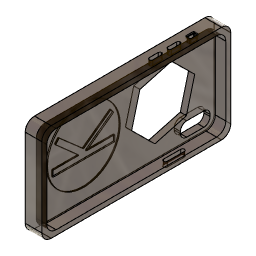
Mitt Mobildeksel (Autodesk Fusion 360 design; units mm, degrees)
Autodesk Fusion 360 part; units mm, degrees
sketch "Sketch1" plane through (0, 0, 0) normal (1, 0, 0) x (0, 1, 0)
  line L0 (76.5, 39.5) -> (-76.5, 39.5)
  line L1 (-76.5, 39.5) -> (-76.5, -39.5)
  line L2 (-76.5, -39.5) -> (76.5, -39.5)
  line L3 (76.5, -39.5) -> (76.5, 39.5)
  line L4 (76.5, 39.5) -> (-76.5, -39.5) construction
  line L5 (-76.5, 39.5) -> (76.5, -39.5) construction
  dimension "d6" = 153
  dimension "d7" = 79
  constraint horizontal L0
  constraint perpendicular L0 L1
  constraint parallel L0 L2
  constraint parallel L1 L3
  constraint coincident L4 origin
  constraint coincident L5 origin
  measures "d6" distance of L1.end L2.end
  measures "d7" distance of L0.end L1.end
extrude "Extrude1" add sketch "Sketch1" along normal blind 13.5
sketch "Sketch2" plane through (0, 0, 0) normal (1, 0, 0) x (0, 1, 0)
sketch "Sketch3" plane through (13.5, 0, 0) normal (1, 0, 0) x (0, 1, 0)
  line L0 (76.5, -39.5) -> (76.5, 39.5)
  line L1 (76.5, 39.5) -> (-76.5, 39.5)
  line L2 (-76.5, 39.5) -> (-76.5, -39.5)
  line L3 (-76.5, -39.5) -> (76.5, -39.5)
  line L4 (72.5, 35.5) -> (-72.5, 35.5)
  line L5 (-72.5, 35.5) -> (-72.5, -35.5)
  line L6 (-72.5, -35.5) -> (72.5, -35.5)
  line L7 (72.5, -35.5) -> (72.5, 35.5)
  line L8 (72.5, 35.5) -> (-72.5, -35.5) construction
  line L9 (-72.5, 35.5) -> (72.5, -35.5) construction
  dimension "d10" = 145
  dimension "d11" = 71
  constraint horizontal L4
  constraint perpendicular L4 L5
  constraint parallel L4 L6
  constraint parallel L5 L7
  constraint coincident L8 origin
  constraint coincident L9 origin
  measures "d10" distance of L5.end L6.end
  measures "d11" distance of L4.end L5.end
extrude "Extrude2" cut sketch "Sketch3" against normal blind 8.5 contours L4 L5 L6 L7
fillet "Fillet1" radius 7.5 4 edges at (6.75, -76.5, 39.5) (6.75, 76.5, 39.5) (6.75, -76.5, -39.5) (6.75, 76.5, -39.5)
fillet "Fillet2" radius 7.5 4 edges at (9.25, -72.5, 35.5) (9.25, 72.5, -35.5) (9.25, 72.5, 35.5) (9.25, -72.5, -35.5)
sketch "Sketch4" plane through (0, 0, 0) normal (-1, 0, 0) x (0, -1, 0)
  arc A0 (-76.5, -32) -> (-69, -39.5) centre (-69, -32) ccw
  line L0 (-69, -39.5) -> (69, -39.5)
  arc A1 (69, -39.5) -> (76.5, -32) centre (69, -32) ccw
  line L1 (76.5, -32) -> (76.5, 32)
  arc A2 (76.5, 32) -> (69, 39.5) centre (69, 32) ccw
  line L2 (69, 39.5) -> (-69, 39.5)
  arc A3 (-69, 39.5) -> (-76.5, 32) centre (-69, 32) ccw
  line L3 (-76.5, 32) -> (-76.5, -32)
  line L4 (-44.2147, -20.46) -> (-68.2147, -20.46)
  line L5 (-68.2147, -20.46) -> (-68.2147, -31.96)
  line L6 (-68.2147, -31.96) -> (-44.2147, -31.96)
  line L7 (-44.2147, -31.96) -> (-44.2147, -20.46)
  line L8 (-44.2147, -20.46) -> (-68.2147, -31.96) construction
  line L9 (-68.2147, -20.46) -> (-44.2147, -31.96) construction
  point P0 (-56.2147, -26.21)
  dimension "d16" = 24
  dimension "d17" = 11.5
  constraint horizontal L4
  constraint perpendicular L4 L5
  constraint parallel L4 L6
  constraint parallel L5 L7
  constraint coincident L8 P0
  constraint coincident L9 P0
  measures "d16" distance of L5.end L6.end
  measures "d17" distance of L4.end L5.end
extrude "Extrude3" cut sketch "Sketch4" against normal blind 20 contours L4 L5 L6 L7
fillet "Fillet3" radius 5 4 edges at (2.5, 44.2147, -20.46) (2.5, 68.2147, -20.46) (2.5, 44.2147, -31.96) (2.5, 68.2147, -31.96)
sketch "Sketch5" plane through (0, 0, -35.5) normal (0, 0, 1) x (-1, 0, 0)
  line L0 (-5, 65) -> (-13.5, 65)
  line L1 (-13.5, 65) -> (-13.5, -65)
  line L2 (-13.5, -65) -> (-5, -65)
  line L3 (-5, -65) -> (-5, 65)
  line L4 (-7.5, -26.5) -> (-10.5, -26.5)
  line L5 (-10.5, -26.5) -> (-10.5, -43.5)
  line L6 (-10.5, -43.5) -> (-7.5, -43.5)
  line L7 (-7.5, -43.5) -> (-7.5, -26.5)
  line L8 (-7.5, -26.5) -> (-10.5, -43.5) construction
  line L9 (-10.5, -26.5) -> (-7.5, -43.5) construction
  point P0 (-9, -35)
  dimension "d21" = 3
  dimension "d22" = 17
  constraint horizontal L4
  constraint perpendicular L4 L5
  constraint parallel L4 L6
  constraint parallel L5 L7
  constraint coincident L8 P0
  constraint coincident L9 P0
  measures "d21" distance of L5.end L6.end
  measures "d22" distance of L4.end L5.end
extrude "Extrude4" cut sketch "Sketch5" against normal blind 6 contours L4 L5 L6 L7
fillet "Fillet4" radius 1.5 4 edges at (7.5, 26.5, -37.5) (10.5, 26.5, -37.5) (7.5, 43.5, -37.5) (10.5, 43.5, -37.5)
sketch "Sketch6" plane through (0, 0, 39.5) normal (0, 0, 1) x (-1, 0, 0)
  line L0 (-13.5, -69) -> (0, -69)
  line L1 (0, -69) -> (0, 69)
  line L2 (0, 69) -> (-13.5, 69)
  line L3 (-13.5, 69) -> (-13.5, -69)
  line L4 (-8.5982, -48.5986) -> (-5.5982, -48.5986)
  line L5 (-5.5982, -48.5986) -> (-5.5982, -54.5986)
  line L6 (-5.5982, -54.5986) -> (-8.5982, -54.5986)
  line L7 (-8.5982, -54.5986) -> (-8.5982, -48.5986)
  line L8 (-8.5982, -48.5986) -> (-5.5982, -54.5986) construction
  line L9 (-5.5982, -48.5986) -> (-8.5982, -54.5986) construction
  point P0 (-7.0982, -51.5986)
  dimension "d26" = 3
  dimension "d27" = 6
  constraint horizontal L4
  constraint perpendicular L4 L5
  constraint parallel L4 L6
  constraint parallel L5 L7
  constraint coincident L8 P0
  constraint coincident L9 P0
  measures "d26" distance of L5.end L6.end
  measures "d27" distance of L4.end L5.end
extrude "Extrude5" cut sketch "Sketch6" against normal blind 5 contours L4 L5 L6 L7
sketch "Sketch7" plane through (0, 0, 39.5) normal (0, 0, 1) x (-1, 0, 0)
  line L0 (-5.5982, -48.5986) -> (-5.5982, -54.5986)
  line L1 (-5.5982, -54.5986) -> (-8.5982, -54.5986)
  line L2 (-8.5982, -54.5986) -> (-8.5982, -48.5986)
  line L3 (-8.5982, -48.5986) -> (-5.5982, -48.5986)
  line L4 (-13.5, -69) -> (0, -69)
  line L5 (0, -69) -> (0, 69)
  line L6 (0, 69) -> (-13.5, 69)
  line L7 (-13.5, 69) -> (-13.5, -69)
  line L8 (-9, -48.3) -> (-5, -48.3)
  line L9 (-5, -48.3) -> (-5, -54.9)
  line L10 (-5, -54.9) -> (-9, -54.9)
  line L11 (-9, -54.9) -> (-9, -48.3)
  line L12 (-9, -48.3) -> (-5, -54.9) construction
  line L13 (-5, -48.3) -> (-9, -54.9) construction
  point P0 (-7, -51.6)
  constraint horizontal L8
  constraint perpendicular L8 L9
  constraint parallel L8 L10
  constraint parallel L9 L11
  constraint coincident L12 P0
  constraint coincident L13 P0
extrude "Extrude6" cut sketch "Sketch7" against normal blind 1 contours L8 L9 L10 L11
fillet "Fillet5" radius 0.5 4 edges at (5.5982, 54.5986, 37) (8.5982, 48.5986, 37) (5.5982, 48.5986, 37) (8.5982, 54.5986, 37)
fillet "Fillet6" radius 0.5 4 edges at (9, 54.9, 39) (9, 48.3, 39) (5, 48.3, 39) (5, 54.9, 39)
sketch "Sketch8" plane through (0, 0, 39.5) normal (0, 0, 1) x (-1, 0, 0)
  line L0 (-5, -48.8) -> (-5, -54.4)
  arc A0 (-5.5, -54.9) -> (-5, -54.4) centre (-5.5, -54.4) ccw
  line L1 (-5.5, -54.9) -> (-8.5, -54.9)
  arc A1 (-9, -54.4) -> (-8.5, -54.9) centre (-8.5, -54.4) ccw
  line L2 (-9, -54.4) -> (-9, -48.8)
  arc A2 (-8.5, -48.3) -> (-9, -48.8) centre (-8.5, -48.8) ccw
  line L3 (-8.5, -48.3) -> (-5.5, -48.3)
  arc A3 (-5, -48.8) -> (-5.5, -48.3) centre (-5.5, -48.8) ccw
  line L4 (-13.5, -69) -> (0, -69)
  line L5 (0, -69) -> (0, 69)
  line L6 (0, 69) -> (-13.5, 69)
  line L7 (-13.5, 69) -> (-13.5, -69)
  line L8 (-5.5, -42) -> (-8.5, -42)
  line L9 (-8.5, -42) -> (-8.5, -32)
  line L10 (-8.5, -32) -> (-5.5, -32)
  line L11 (-5.5, -32) -> (-5.5, -42)
  line L12 (-5.5, -42) -> (-8.5, -32) construction
  line L13 (-8.5, -42) -> (-5.5, -32) construction
  point P0 (-7, -37)
  dimension "d34" = 3
  dimension "d35" = 10
  constraint horizontal L8
  constraint perpendicular L8 L9
  constraint parallel L8 L10
  constraint parallel L9 L11
  constraint coincident L12 P0
  constraint coincident L13 P0
  measures "d34" distance of L9.end L10.end
  measures "d35" distance of L8.end L9.end
extrude "Extrude7" cut sketch "Sketch8" against normal blind 17 contours L8 L9 L10 L11
sketch "Sketch9" plane through (0, 0, 39.5) normal (0, 0, 1) x (-1, 0, 0)
  line L0 (-8.5, -42) -> (-8.5, -32)
  line L1 (-8.5, -32) -> (-5.5, -32)
  line L2 (-5.5, -32) -> (-5.5, -42)
  line L3 (-5.5, -42) -> (-8.5, -42)
  line L4 (-5, -48.8) -> (-5, -54.4)
  arc A0 (-5.5, -54.9) -> (-5, -54.4) centre (-5.5, -54.4) ccw
  line L5 (-5.5, -54.9) -> (-8.5, -54.9)
  arc A1 (-9, -54.4) -> (-8.5, -54.9) centre (-8.5, -54.4) ccw
  line L6 (-9, -54.4) -> (-9, -48.8)
  arc A2 (-8.5, -48.3) -> (-9, -48.8) centre (-8.5, -48.8) ccw
  line L7 (-8.5, -48.3) -> (-5.5, -48.3)
  arc A3 (-5, -48.8) -> (-5.5, -48.3) centre (-5.5, -48.8) ccw
  line L8 (-13.5, -69) -> (0, -69)
  line L9 (0, -69) -> (0, 69)
  line L10 (0, 69) -> (-13.5, 69)
  line L11 (-13.5, 69) -> (-13.5, -69)
  line L12 (-8.5, -27) -> (-5.5, -27)
  line L13 (-5.5, -27) -> (-5.5, -17)
  line L14 (-5.5, -17) -> (-8.5, -17)
  line L15 (-8.5, -17) -> (-8.5, -27)
  line L16 (-8.5, -27) -> (-5.5, -17) construction
  line L17 (-5.5, -27) -> (-8.5, -17) construction
  point P0 (-7, -22)
  dimension "d38" = 3
  dimension "d39" = 10
  constraint horizontal L12
  constraint perpendicular L12 L13
  constraint parallel L12 L14
  constraint parallel L13 L15
  constraint coincident L16 P0
  constraint coincident L17 P0
  measures "d38" distance of L13.end L14.end
  measures "d39" distance of L12.end L13.end
extrude "Extrude8" cut sketch "Sketch9" against normal blind 9 contours L12 L13 L14 L15
fillet "Fillet7" radius 1.25 4 edges at (5.5, 32, 37.5) (8.5, 32, 37.5) (5.5, 42, 37.5) (8.5, 42, 37.5)
fillet "Fillet8" radius 1.25 4 edges at (8.5, 27, 37.5) (5.5, 27, 37.5) (8.5, 17, 37.5) (5.5, 17, 37.5)
form "Form1" [no effect]
sketch "Sketch10" plane through (0, 0, 0) normal (-1, 0, 0) x (0, -1, 0)
  line L0 (-63.2147, -20.46) -> (-49.2147, -20.46)
  arc A0 (-44.2147, -25.46) -> (-49.2147, -20.46) centre (-49.2147, -25.46) ccw
  line L1 (-44.2147, -25.46) -> (-44.2147, -26.96)
  arc A1 (-49.2147, -31.96) -> (-44.2147, -26.96) centre (-49.2147, -26.96) ccw
  line L2 (-49.2147, -31.96) -> (-63.2147, -31.96)
  arc A2 (-68.2147, -26.96) -> (-63.2147, -31.96) centre (-63.2147, -26.96) ccw
  line L3 (-68.2147, -26.96) -> (-68.2147, -25.46)
  arc A3 (-63.2147, -20.46) -> (-68.2147, -25.46) centre (-63.2147, -25.46) ccw
  arc A4 (-76.5, -32) -> (-69, -39.5) centre (-69, -32) ccw
  line L4 (-69, -39.5) -> (69, -39.5)
  arc A5 (69, -39.5) -> (76.5, -32) centre (69, -32) ccw
  line L5 (76.5, -32) -> (76.5, 32)
  arc A6 (76.5, 32) -> (69, 39.5) centre (69, 32) ccw
  line L6 (69, 39.5) -> (-69, 39.5)
  arc A7 (-69, 39.5) -> (-76.5, 32) centre (-69, 32) ccw
  line L7 (-76.5, 32) -> (-76.5, -32)
  line L8 (-11.3981, 20.5126) -> (-36.9638, 27.5049)
  line L9 (-36.9638, 27.5049) -> (-55.8022, 8.8605)
  line L10 (-55.8022, 8.8605) -> (-49.0748, -16.7762)
  line L11 (-49.0748, -16.7762) -> (-23.5091, -23.7685)
  line L12 (-23.5091, -23.7685) -> (-4.6707, -5.1241)
  line L13 (-4.6707, -5.1241) -> (-11.3981, 20.5126)
  point P0 (-30.2365, 1.8682)
extrude "Extrude9" cut sketch "Sketch10" against normal blind 15 contours L8 L9 L10 L11 L12 L13
sketch "Sketch11" plane through (0, 0, 0) normal (-1, 0, 0) x (0, -1, 0)
  line L0 (-36.9638, 27.5049) -> (-11.3981, 20.5126)
  line L1 (-11.3981, 20.5126) -> (-4.6707, -5.1241)
  line L2 (-4.6707, -5.1241) -> (-23.5091, -23.7685)
  line L3 (-23.5091, -23.7685) -> (-49.0748, -16.7762)
  line L4 (-49.0748, -16.7762) -> (-55.8022, 8.8605)
  line L5 (-55.8022, 8.8605) -> (-36.9638, 27.5049)
  line L6 (-63.2147, -20.46) -> (-49.2147, -20.46)
  arc A0 (-44.2147, -25.46) -> (-49.2147, -20.46) centre (-49.2147, -25.46) ccw
  line L7 (-44.2147, -25.46) -> (-44.2147, -26.96)
  arc A1 (-49.2147, -31.96) -> (-44.2147, -26.96) centre (-49.2147, -26.96) ccw
  line L8 (-49.2147, -31.96) -> (-63.2147, -31.96)
  arc A2 (-68.2147, -26.96) -> (-63.2147, -31.96) centre (-63.2147, -26.96) ccw
  line L9 (-68.2147, -26.96) -> (-68.2147, -25.46)
  arc A3 (-63.2147, -20.46) -> (-68.2147, -25.46) centre (-63.2147, -25.46) ccw
  arc A4 (-76.5, -32) -> (-69, -39.5) centre (-69, -32) ccw
  line L10 (-69, -39.5) -> (69, -39.5)
  arc A5 (69, -39.5) -> (76.5, -32) centre (69, -32) ccw
  line L11 (76.5, -32) -> (76.5, 32)
  arc A6 (76.5, 32) -> (69, 39.5) centre (69, 32) ccw
  line L12 (69, 39.5) -> (-69, 39.5)
  arc A7 (-69, 39.5) -> (-76.5, 32) centre (-69, 32) ccw
  line L13 (-76.5, 32) -> (-76.5, -32)
  circle A8 centre (30, 0) radius 29.4535
extrude "Extrude10" add sketch "Sketch11" along normal blind 1 contours A8
extrude "Extrude11" cut 1 faces at (-1, -23.9019, 17.2803) along direction (1, 0, 0) blind 2
sketch "Sketch12" plane through (1, 0, 0) normal (-1, 0, 0) x (0, -1, 0)
  circle A0 centre (30, 0) radius 29.4535
  line L0 (5, -10) -> (55, -10)
  line L1 (55, -10) -> (55, -5)
  line L2 (55, -5) -> (5, -5)
  line L3 (5, -5) -> (5, -10)
  line L4 (25, -5) -> (7.4976, 11.068)
  line L5 (7.4976, 11.068) -> (10.2461, 14.0619)
  line L6 (10.2461, 14.0619) -> (31.0096, -5)
  line L7 (35, -5) -> (52.8189, 12.5649)
  line L8 (52.8189, 12.5649) -> (50.2221, 15.1993)
  line L9 (50.2221, 15.1993) -> (30.3474, -4.3921)
  constraint horizontal L0
  constraint perpendicular L0 L1
  constraint perpendicular L1 L2
  constraint perpendicular L0 L3
  constraint coincident L2 L4.start
  constraint perpendicular L4 L5
  constraint coincident L2 L6.end
  constraint perpendicular L5 L6
  constraint coincident L2 L7.start
  constraint perpendicular L7 L8
  constraint coincident L6 L9.end
  constraint perpendicular L8 L9
extrude "Extrude12" add sketch "Sketch12" along normal blind 1 contours L0 L1 L2 L3
sketch "Sketch13" plane through (1, 0, 0) normal (-1, 0, 0) x (0, -1, 0)
  line L0 (5, -5) -> (55, -5)
  line L1 (55, -5) -> (55, -10)
  line L2 (55, -10) -> (5, -10)
  line L3 (5, -10) -> (5, -5)
  circle A0 centre (30, 0) radius 29.4535
  line L4 (27.8903, -5) -> (5.8744, 11.0918)
  line L5 (5.8744, 11.0918) -> (8, 14)
  line L6 (8, 14) -> (33.9947, -5)
  constraint coincident L0 L4.start
  constraint perpendicular L4 L5
  constraint coincident L0 L6.end
  constraint perpendicular L5 L6
extrude "Extrude13" add sketch "Sketch13" along normal blind 1 contours L0 L4 L5 L6
sketch "Sketch14" plane through (1, 0, 0) normal (-1, 0, 0) x (0, -1, 0)
  circle A0 centre (30, 0) radius 29.4535
  line L0 (27.8903, -5) -> (5.8744, 11.0918)
  line L1 (5.8744, 11.0918) -> (8, 14)
  line L2 (8, 14) -> (33.9947, -5)
  line L3 (33.9947, -5) -> (55, -5)
  line L4 (55, -5) -> (55, -10)
  line L5 (55, -10) -> (5, -10)
  line L6 (5, -10) -> (5, -5)
  line L7 (5, -5) -> (27.8903, -5)
  line L8 (30.2858, -2.2891) -> (50, 15)
  line L9 (50, 15) -> (52.8643, 11.7339)
  line L10 (52.8643, 11.7339) -> (33.9947, -5)
  constraint coincident L2 L8.start
  constraint perpendicular L8 L9
  constraint coincident L2.end L3.start
extrude "Extrude14" add sketch "Sketch14" along normal blind 1 contours L2 L8 L9 L10
equation "høyde = 145 mm"
equation "bredde = 71 mm"
equation "tykkelse = 8.5 mm"
equation "kamerahøyde = 24 mm"
equation "kamerabredde = 11.5 mm"
equation "d6 = høyde + 8 mm"
equation "d7 = bredde + 8 mm"
equation "d8 = tykkelse + 5 mm"
equation "d10 = høyde"
equation "d11 = bredde"
equation "d12 = -tykkelse"
equation "d16 = kamerahøyde"
equation "d17 = kamerabredde"
